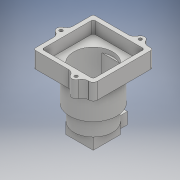
# Autodesk Inventor part: Dubmmy
Saved by Autodesk Inventor 2017 (Build 210142000, 142)
## iProperties
Created: 2017-12-13
Part Number: Dubmmy
Material: Generic
Document SubType Name: Modeling
Designer: andrew
Density: 1 g/cm^3
Appearance: Default
Author: andrew
Autodesk Inventor part; units mm, degrees
ref_plane "YZ Plane" through (0, 0, 0) normal (1, 0, 0) x (0, 1, 0)
ref_plane "XZ Plane" through (0, 0, 0) normal (0, 1, 0) x (-1, 0, 0)
ref_plane "XY Plane" through (0, 0, 0) normal (0, 0, 1) x (1, 0, 0)
sketch "Sketch1" plane through (0, 0, 0) normal (0, 0, 1) x (1, 0, 0)
  arc A0 (-2.0222, 4.0759) -> (2.0222, 4.0759) centre (0, 0) ccw
  circle A1 centre (0, 0) radius 5.5
  line L0 (2.0222, 4.0759) -> (-2.0222, 4.0759)
  dimension "d0" = 11
  dimension "d45" = 4.55
  constraints: 2 centre point, 2 end point, 2 point on circle
  measures "d0" diameter of A1
  measures "d45" radius of A0
extrude "Extrusion1" add sketch "Sketch1" along normal blind 7
sketch "Sketch2" plane through (0, 0, 0) normal (0, 0, -1) x (-1, 0, 0)
  line L0 (-1.25, 5.125) -> (1.25, 5.125) construction
  circle A0 centre (0, 0) radius 5.5 construction
  line L1 (0, 0) -> (0, 9.5083) construction
  circle A1 centre (0, 0) radius 5.5 construction
  line L2 (0, 5.5) -> (0, 7.7304) construction
  line L3 (0, 5.125) -> (0, 7.5987) construction
  line L4 (-1.25, 5.125) -> (-1.25, 6.125) construction
  line L5 (-1.25, 6.125) -> (1.25, 6.125)
  line L6 (1.25, 6.125) -> (1.25, 4.5986)
  line L7 (1.25, 4.5986) -> (-1.25, 4.5986)
  line L8 (-1.25, 4.5986) -> (-1.25, 6.125)
  dimension "d3" = 2.5
  dimension "d4" = 1
  constraints: 18 end point, 3 vertical, 2 horizontal, 2 parallel, 2 point on line, 1 midpoint, 1 perpendicular, 1 vertical alignment, 1 other
  measures "d3" distance of L0.start L0.end
  measures "d4" distance of L0.start L4.end
extrude "Extrusion2" add sketch "Sketch2" against normal blind 5
sketch "Sketch3" plane through (0, 0, 7) normal (0, 0, 1) x (1, 0, 0)
  line L0 (7, 6.5) -> (7, -6)
  arc A0 (6, -7) -> (7, -6) centre (6, -6) ccw
  arc A1 (-7, -6.5) -> (-6.5, -7) centre (-6.5, -6.5) ccw
  arc A2 (-6.5, 7) -> (-7, 6.5) centre (-6.5, 6.5) ccw
  arc A3 (7, 6.5) -> (6.5, 7) centre (6.5, 6.5) ccw
  line L1 (6, -5.5) -> (6, 5.5)
  line L2 (5.5, 6) -> (-5.5, 6)
  line L3 (-6, 5.5) -> (-6, -5.5)
  line L4 (-5.5, -6) -> (5.5, -6)
  arc A4 (5.5, -6) -> (6, -5.5) centre (5.5, -5.5) ccw
  arc A5 (6, 5.5) -> (5.5, 6) centre (5.5, 5.5) ccw
  arc A6 (-5.5, 6) -> (-6, 5.5) centre (-5.5, 5.5) ccw
  arc A7 (-6, -5.5) -> (-5.5, -6) centre (-5.5, -5.5) ccw
  line L5 (8.9739, -10.9736) -> (8.9739, -4.3472) construction
  arc A8 (2.5835, -7.9) -> (4.4165, -7.9) centre (3.5, -7.5) ccw
  circle A9 centre (3.5, -7.5) radius 0.375
  arc A10 (-7.9, 0.9165) -> (-7.9, -0.9165) centre (-7.5, 0) ccw
  circle A11 centre (-7.5, 0) radius 0.375
  arc A12 (4.4165, 7.9) -> (2.5835, 7.9) centre (3.5, 7.5) ccw
  circle A13 centre (3.5, 7.5) radius 0.375
  line L6 (6, -7) -> (5.7913, -7)
  line L7 (1.2087, -7) -> (-6.5, -7)
  arc A14 (5.7913, -7) -> (4.4165, -7.9) centre (5.7913, -8.5) ccw
  arc A15 (2.5835, -7.9) -> (1.2087, -7) centre (1.2087, -8.5) ccw
  line L8 (-7, -6.5) -> (-7, -2.2913)
  line L9 (-7, 2.2913) -> (-7, 6.5)
  arc A16 (-7, -2.2913) -> (-7.9, -0.9165) centre (-8.5, -2.2913) ccw
  arc A17 (-7.9, 0.9165) -> (-7, 2.2913) centre (-8.5, 2.2913) ccw
  line L10 (-6.5, 7) -> (1.2087, 7)
  line L11 (5.7913, 7) -> (6.5, 7)
  arc A18 (4.4165, 7.9) -> (5.7913, 7) centre (5.7913, 8.5) ccw
  arc A19 (1.2087, 7) -> (2.5835, 7.9) centre (1.2087, 8.5) ccw
  arc A20 (-2.0222, 4.0759) -> (2.0222, 4.0759) centre (0, 0) ccw projected
  circle A21 centre (0, 0) radius 4.55
  point P0 (-7, 7)
  point P1 (-7, -7)
  point P2 (7, 7)
  point P3 (4.366, -7)
  point P4 (2.634, -7)
  point P5 (-7, -0.866)
  point P6 (-7, 0.866)
  point P7 (2.634, 7)
  point P8 (4.366, 7)
  point P9 (1, 4.3875)
  point P10 (-1, 4.3875)
  dimension "d9" = 14
  dimension "d11" = 1
  dimension "d13" = 1
  dimension "d14" = 0.5
  dimension "d15" = 2
  dimension "d16" = 0.75
  dimension "d18" = 0.75
  dimension "d19" = 2
  dimension "d20" = 0.75
  dimension "d21" = 1.5
  dimension "d22" = 1.5
  dimension "d23" = 1.5
  constraints: 40 point on circle, 34 tangent, 24 end point, 21 centre point, 8 equal radius, 8 parallel, 7 coincident, 7 point on line, 5 perpendicular, 2 horizontal, 1 vertical, 2 other
  measures "d9" distance of point (-7, 7) point (7, 7)
  measures "d11" radius of A0
  measures "d13" distance between parallel lines of L0 L1
  measures "d14" radius of A4
  measures "d15" diameter of A8
  measures "d16" diameter of A9
  measures "d18" diameter of A11
  measures "d19" diameter of A12
  measures "d20" diameter of A13
  measures "d21" radius of A14
  measures "d22" radius of A16
  measures "d23" radius of A18
extrude "Extrusion3" add sketch "Sketch3" along normal blind 1 contours L0 A0 L6 A14 A8 A15 L7 A1 L8 A16 A10 A17 L9 A2 L10 A19 A12 A18 L11 A3 | A4 L4 A7 L3 A6 L2 A5 L1
sketch "Sketch4" plane through (0, 0, 8) normal (0, 0, 1) x (1, 0, 0)
  line L0 (7, 6.5) -> (7, -6)
  arc A0 (6, -7) -> (7, -6) centre (6, -6) ccw
  arc A1 (-7, -6.5) -> (-6.5, -7) centre (-6.5, -6.5) ccw
  arc A2 (-6.5, 7) -> (-7, 6.5) centre (-6.5, 6.5) ccw
  arc A3 (7, 6.5) -> (6.5, 7) centre (6.5, 6.5) ccw
  line L1 (6, -5.5) -> (6, 5.5)
  line L2 (5.5, 6) -> (-5.5, 6)
  line L3 (-6, 5.5) -> (-6, -5.5)
  line L4 (-5.5, -6) -> (5.5, -6)
  arc A4 (5.5, -6) -> (6, -5.5) centre (5.5, -5.5) ccw
  arc A5 (6, 5.5) -> (5.5, 6) centre (5.5, 5.5) ccw
  arc A6 (-5.5, 6) -> (-6, 5.5) centre (-5.5, 5.5) ccw
  arc A7 (-6, -5.5) -> (-5.5, -6) centre (-5.5, -5.5) ccw
  line L5 (8.9739, -10.9736) -> (8.9739, -4.3472) construction
  arc A8 (2.5835, -7.9) -> (4.4165, -7.9) centre (3.5, -7.5) ccw
  circle A9 centre (3.5, -7.5) radius 0.375
  arc A10 (-7.9, 0.9165) -> (-7.9, -0.9165) centre (-7.5, 0) ccw
  circle A11 centre (-7.5, 0) radius 0.375
  arc A12 (4.4165, 7.9) -> (2.5835, 7.9) centre (3.5, 7.5) ccw
  circle A13 centre (3.5, 7.5) radius 0.375
  line L6 (6, -7) -> (5.7913, -7)
  line L7 (1.2087, -7) -> (-6.5, -7)
  arc A14 (5.7913, -7) -> (4.4165, -7.9) centre (5.7913, -8.5) ccw
  arc A15 (2.5835, -7.9) -> (1.2087, -7) centre (1.2087, -8.5) ccw
  line L8 (-7, -6.5) -> (-7, -2.2913)
  line L9 (-7, 2.2913) -> (-7, 6.5)
  arc A16 (-7, -2.2913) -> (-7.9, -0.9165) centre (-8.5, -2.2913) ccw
  arc A17 (-7.9, 0.9165) -> (-7, 2.2913) centre (-8.5, 2.2913) ccw
  line L10 (-6.5, 7) -> (1.2087, 7)
  line L11 (5.7913, 7) -> (6.5, 7)
  arc A18 (4.4165, 7.9) -> (5.7913, 7) centre (5.7913, 8.5) ccw
  arc A19 (1.2087, 7) -> (2.5835, 7.9) centre (1.2087, 8.5) ccw
  arc A20 (-1, 4.3875) -> (1, 4.3875) centre (0, 0) ccw
  circle A21 centre (0, 0) radius 4.5
  point P0 (-7, 7)
  point P1 (-7, -7)
  point P2 (7, 7)
  point P3 (4.366, -7)
  point P4 (2.634, -7)
  point P5 (-7, -0.866)
  point P6 (-7, 0.866)
  point P7 (2.634, 7)
  point P8 (4.366, 7)
  dimension "d26" = 14
  dimension "d27" = 1
  dimension "d28" = 1
  dimension "d29" = 0.5
  dimension "d30" = 2
  dimension "d31" = 0.75
  dimension "d32" = 0.75
  dimension "d33" = 2
  dimension "d34" = 0.75
  dimension "d35" = 1.5
  dimension "d36" = 1.5
  dimension "d37" = 1.5
  constraints: 42 point on circle, 34 tangent, 24 end point, 22 centre point, 9 equal radius, 8 parallel, 7 coincident, 7 point on line, 5 perpendicular, 2 horizontal, 1 vertical
  measures "d26" distance of point (-7, 7) point (7, 7)
  measures "d27" radius of A0
  measures "d28" distance between parallel lines of L0 L1
  measures "d29" radius of A4
  measures "d30" diameter of A8
  measures "d31" diameter of A9
  measures "d32" diameter of A11
  measures "d33" diameter of A12
  measures "d34" diameter of A13
  measures "d35" radius of A14
  measures "d36" radius of A16
  measures "d37" radius of A18
extrude "Extrusion4" add sketch "Sketch4" along normal blind 2.8 contours L0 A0 L6 A14 A8 A15 L7 A1 L8 A16 A10 A17 L9 A2 L10 A19 A12 A18 L11 A3
sketch "Sketch5" plane through (-1.25, 6.125, 0) normal (0, 1, 0) x (1, 0, 0)
  line L0 (1.8283, -3.8925) -> (1.8437, -3.7979)
  line L1 (0.8374, -4.1796) -> (0.9116, -4.2402)
  line L2 (0.7226, -3.4732) -> (0.7738, -3.3922)
  line L3 (1.7534, -0.9317) -> (1.798, -1.0165)
  line L4 (0.8374, -1.6796) -> (0.9116, -1.7402)
  line L5 (0.7738, -0.8922) -> (0.8374, -0.8204)
  line L6 (0, 0) -> (2.5, 0)
  line L7 (0, 0) -> (0, -5)
  circle A0 centre (1.25, -1.25) radius 0.5937
  circle A1 centre (1.25, -3.75) radius 0.5937
  point P0 (1.25, 0)
  point P1 (1.0843, -1.8221)
  dimension "d40" = 1.1874
  constraints: 16 end point, 6 tangent, 2 centre point
  measures "d40" diameter of A1
extrude "Extrusion5" cut sketch "Sketch5" against normal blind 5
fillet "Fillet1" radius 2 2 edges at (-1.25, 5.3561, 2.5) (1.25, 5.3561, 2.5)
chamfer "Chamfer1" distance 0.5 angle 45 2 edges at (0, -4.55, 0) (0, 4.0759, 0)
sketch "Sketch6" plane through (0, 0, 0) normal (0, 0, -1) x (-1, 0, 0)
  arc A0 (-2.2927, 4.9994) -> (2.2927, 4.9994) centre (0, 0) ccw projected
  circle A1 centre (0, 0) radius 5.5
  arc A2 (-3.2581, 3.104) -> (2, 4.0311) centre (0, 0) ccw
  arc A3 (-1.2449, 0.0939) -> (1.2449, 0.0939) centre (0, 0) ccw
  arc A4 (-2.1362, 4.5759) -> (2.1362, 4.5759) centre (0, 0) ccw projected
  circle A5 centre (0, 0) radius 5.05
  circle A6 centre (0, 0) radius 4.5
  circle A7 centre (0, 0) radius 3.5
  dimension "d50" = 7
  constraints: 5 centre point, 4 coincident, 4 point on circle, 2 concentric, 3 other
  measures "d50" diameter of A7
extrude "Extrusion6" add sketch "Sketch6" against normal blind 1 contours A6 A2 | A5 A4
sketch "Sketch7" plane through (0, 0, 0) normal (0, 0, -1) x (-1, 0, 0)
  arc A0 (-2.2927, 4.9994) -> (2.2927, 4.9994) centre (0, 0) ccw
  circle A1 centre (0, 0) radius 5.5
  arc A2 (-3.2581, 3.104) -> (2, 4.0311) centre (0, 0) ccw
  arc A3 (-1.2449, 0.0939) -> (1.2449, 0.0939) centre (0, 0) ccw
  arc A4 (-2.1362, 4.5759) -> (2.1362, 4.5759) centre (0, 0) ccw
  circle A5 centre (0, 0) radius 5.05
  circle A6 centre (0, 0) radius 4.5
  circle A7 centre (0, 0) radius 3.5
  dimension "d53" = 7
  constraints: 8 point on circle, 7 centre point, 4 coincident, 2 concentric, 3 other
  measures "d53" diameter of A7
extrude "Extrusion7" add sketch "Sketch7" along normal blind 3.81 contours A6 A2
sketch "Sketch8" plane through (0, 0, -3.81) normal (0, 0, -1) x (-1, 0, 0)
  line L0 (3.7674, 2.461) -> (4.3315, 3.068)
  line L1 (4.3315, 3.068) -> (2.5, 4.7697)
  line L2 (2.5, 4.7697) -> (2.94, 6)
  line L3 (2.94, 6) -> (-2, 6)
  line L4 (-2, 6) -> (-2, 4.0311)
  arc A0 (-2, 4.0311) -> (-3.182, 3.182) centre (0, 0) ccw
  line L5 (-3.182, 3.182) -> (-3.182, -3.182)
  line L6 (-3.182, -3.182) -> (3.182, -3.182)
  arc A1 (3.182, -3.182) -> (3.7674, 2.461) centre (0, 0) ccw
  circle A2 centre (0, 0) radius 1.2484
  circle A3 centre (0, 3) radius 0.7934
  circle A4 centre (1.875, -1.75) radius 0.7934
  circle A5 centre (-1.875, -1.75) radius 0.7934
  constraints: 14 end point, 6 centre point, 4 point on circle
extrude "Extrusion8" add sketch "Sketch8" along normal blind 1.5 contours A1 L6 L5 A0 L4 L3 L2 L1 L0 | A3 | A4 | A5
sketch "Sketch9" plane through (0, 0, -5.31) normal (0, 0, -1) x (-1, 0, 0)
  line L0 (3.7674, 2.461) -> (4.3315, 3.068)
  line L1 (4.3315, 3.068) -> (2.5, 4.7697)
  line L2 (2.5, 4.7697) -> (2.94, 6)
  line L3 (2.94, 6) -> (-2, 6)
  line L4 (-2, 6) -> (-2, 4.0311)
  arc A0 (-2, 4.0311) -> (-3.182, 3.182) centre (0, 0) ccw
  line L5 (-3.182, 3.182) -> (-3.182, -3.182)
  line L6 (-3.182, -3.182) -> (3.182, -3.182)
  arc A1 (3.182, -3.182) -> (3.7674, 2.461) centre (0, 0) ccw
  circle A2 centre (0, 0) radius 1.2484
  circle A3 centre (0, 3) radius 0.7934
  circle A4 centre (1.875, -1.75) radius 0.7934
  circle A5 centre (-1.875, -1.75) radius 0.7934
  constraints: 14 end point, 6 centre point, 4 point on circle
extrude "Extrusion9" add sketch "Sketch9" along normal blind 1.182
body "Solid1"
